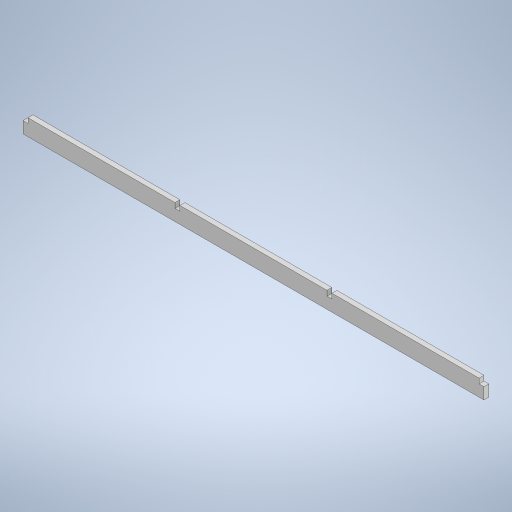
# Autodesk Inventor part: 支撐架
Saved by Autodesk Inventor 2023 (Build 270158000, 158)
## iProperties
Created: 2023-03-24
Part Number: 支撐架
Material: 一般
Document SubType Name: Modeling
Designer: USER
Density: 1 g/cm^3
Appearance: 預設
Author: USER
Autodesk Inventor part; units mm, degrees
ref_plane "YZ Plane" through (0, 0, 0) normal (1, 0, 0) x (0, 1, 0)
ref_plane "XZ Plane" through (0, 0, 0) normal (0, 1, 0) x (-1, 0, 0)
ref_plane "XY Plane" through (0, 0, 0) normal (0, 0, 1) x (1, 0, 0)
sketch "草圖1" plane through (0, 0, 0) normal (0, 0, 1) x (1, 0, 0)
  line L0 (0, 0) -> (280, 0)
  line L1 (280, 0) -> (280, 10)
  line L2 (280, 10) -> (0, 10)
  line L3 (0, 10) -> (0, 0)
  dimension "d0" = 10
  dimension "d1" = 280
  constraints: 8 end point, 2 parallel, 1 horizontal, 1 perpendicular
  measures "d0" distance of L2.end L0.start
  measures "d1" distance of L1.end L2.end
extrude "擠出1" add sketch "草圖1" along normal blind 3
sketch "草圖2" plane through (0, 0, 3) normal (0, 0, 1) x (1, 0, 0)
  line L0 (280, 0) -> (280, 10) projected
  line L1 (280, 10) -> (0, 10) projected
  line L2 (0, 10) -> (0, 0) projected
  line L3 (0, 0) -> (280, 0) projected
  line L4 (0, 10) -> (3, 10)
  line L5 (3, 10) -> (3, 7)
  line L6 (3, 7) -> (0, 7)
  line L7 (0, 7) -> (0, 10)
  line L8 (92.3333, 10) -> (95.3333, 10)
  line L9 (95.3333, 10) -> (95.3333, 7)
  line L10 (95.3333, 7) -> (92.3333, 7)
  line L11 (92.3333, 7) -> (92.3333, 10)
  line L12 (280, 10) -> (277, 10)
  line L13 (277, 10) -> (277, 7)
  line L14 (277, 7) -> (280, 7)
  line L15 (280, 7) -> (280, 10)
  line L16 (184.6667, 10) -> (187.6667, 10)
  line L17 (187.6667, 10) -> (187.6667, 7)
  line L18 (187.6667, 7) -> (184.6667, 7)
  line L19 (184.6667, 7) -> (184.6667, 10)
  point P0 (0, 7)
  dimension "d4" = 3
  dimension "d6" = 89.3333
  dimension "d7" = 89.3333
  dimension "d8" = 7
  dimension "d9" = 10
  constraints: 32 end point, 8 parallel, 6 equal length, 4 horizontal, 4 perpendicular, 2 point on line
  measures "d4" distance of L5.end L6.end
  measures "d6" distance between parallel lines of L11 L5
  measures "d7" distance between parallel lines of L19 L9
  measures "d8" distance between parallel lines of L3 L6
  measures "d9" distance between parallel lines of L3 L16
extrude "擠出2" cut sketch "草圖2" against normal through all contours L14 L13 L1 L0 | L2 L1 L5 L6 | L17 L18 L19 L1 | L1 L9 L10 L11
equation "\"d7\" = d6"
